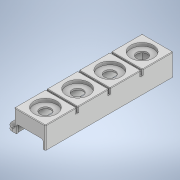
# Autodesk Inventor part: Knob_Base
Saved by Autodesk Inventor 2021 (Build 250183000, 183)
## iProperties
Created: 2020-07-22
Part Number: Knob_Base
Material: Generic
Document SubType Name: Modeling
Designer: ameli
Density: 1 g/cm^3
Appearance: Default
Author: ameli
Autodesk Inventor part; units mm, degrees
ref_plane "YZ Plane" through (0, 0, 0) normal (1, 0, 0) x (0, 1, 0)
ref_plane "XZ Plane" through (0, 0, 0) normal (0, 1, 0) x (-1, 0, 0)
ref_plane "XY Plane" through (0, 0, 0) normal (0, 0, 1) x (1, 0, 0)
sketch "Sketch1" plane through (0, 0, 0) normal (0, 1, 0) x (-1, 0, 0)
  line L0 (14.5, 59.5) -> (-14.5, 59.5)
  line L1 (-14.5, 59.5) -> (-14.5, -59.5)
  line L2 (-14.5, -59.5) -> (14.5, -59.5)
  line L3 (14.5, -59.5) -> (14.5, 59.5)
  point P0 (0, 0)
  dimension "d0" = 119
  dimension "d1" = 29
  dimension "d2" = 14.5
  dimension "d3" = 59.5
  constraints: 8 end point, 2 parallel, 1 horizontal, 1 perpendicular
  measures "d0" distance of L2.end L0.start
  measures "d1" distance of L1.end L2.end
  measures "d2" distance from line of point (0, 0) L3
  measures "d3" distance from line of point (0, 0) L2
extrude "Extrusion1" add sketch "Sketch1" along normal blind 20.3
sketch "Sketch2" plane through (0, 20.3, 0) normal (0, 1, 0) x (1, 0, 0)
  circle A0 centre (0, -45) radius 10.5
  circle A1 centre (0, -15) radius 10.5
  circle A2 centre (0, 15) radius 10.5
  circle A3 centre (0, 45) radius 10.5
  line L0 (-14.5, 59.5) -> (-14.5, -59.5) projected
  line L1 (-14.5, -59.5) -> (14.5, -59.5) projected
  line L2 (14.5, 59.5) -> (-14.5, 59.5) projected
  point P0 (0, 0)
  dimension "d9" = 21
  dimension "d10" = 21
  dimension "d11" = 21
  dimension "d12" = 21
  dimension "d13" = 14.5
  dimension "d14" = 14.5
  dimension "d15" = 14.5
  dimension "d16" = 14.5
  dimension "d17" = 14.5
  dimension "d18" = 14.5
  dimension "d19" = 44.5
  dimension "d20" = 44.5
  constraints: 4 centre point
  measures "d9" diameter of A0
  measures "d10" diameter of A1
  measures "d11" diameter of A2
  measures "d12" diameter of A3
  measures "d13" distance from line of L0 A0.centre
  measures "d14" distance from line of L0 A1.centre
  measures "d15" distance from line of L0 A2.centre
  measures "d16" distance from line of L0 A3.centre
  measures "d17" distance from line of L1 A0.centre
  measures "d18" distance from line of A3.centre L2
  measures "d19" distance from line of L1 A1.centre
  measures "d20" distance from line of L2 A2.centre
extrude "Extrusion2" cut sketch "Sketch2" against normal through all
sketch "Sketch3" plane through (0, 20.3, 0) normal (0, 1, 0) x (1, 0, 0)
  line L0 (-14.5, -30.5) -> (14.5, -30.5)
  line L1 (14.5, -30.5) -> (14.5, -29.5)
  line L2 (14.5, -29.5) -> (-14.5, -29.5)
  line L3 (-14.5, -29.5) -> (-14.5, -30.5)
  line L4 (-14.5, -0.5) -> (14.5, -0.5)
  line L5 (14.5, -0.5) -> (14.5, 0.5)
  line L6 (14.5, 0.5) -> (-14.5, 0.5)
  line L7 (-14.5, 0.5) -> (-14.5, -0.5)
  line L8 (-14.5, 29.5) -> (14.5, 29.5)
  line L9 (14.5, 29.5) -> (14.5, 30.5)
  line L10 (14.5, 30.5) -> (-14.5, 30.5)
  line L11 (-14.5, 30.5) -> (-14.5, 29.5)
  line L12 (-14.5, 59.5) -> (-14.5, -59.5) projected
  line L13 (-14.5, -59.5) -> (14.5, -59.5) projected
  point P0 (0, 0)
  dimension "d23" = 1
  dimension "d24" = 1
  dimension "d25" = 1
  dimension "d26" = 29
  dimension "d27" = 0
  dimension "d28" = 0
  dimension "d29" = 29
  dimension "d30" = 29
  dimension "d31" = 29
  dimension "d32" = 29
  dimension "d33" = 29
  constraints: 24 end point, 6 parallel, 3 horizontal, 3 perpendicular, 1 point on line
  measures "d23" distance of L2.end L0.start
  measures "d24" distance of L6.end L4.start
  measures "d25" distance of L10.end L8.start
  measures "d26" distance of L1.end L2.end
  measures "d27" distance between parallel lines of L12 L3
  measures "d28" distance between parallel lines of L12 L11
  measures "d29" distance of L4.start L4.end
  measures "d30" distance of L8.start L8.end
  measures "d31" distance between parallel lines of L13 L0
  measures "d32" distance between parallel lines of L4 L2
  measures "d33" distance between parallel lines of L8 L6
extrude "Extrusion3" cut sketch "Sketch3" against normal blind 5
shell "Shell2" thickness 1.5 removed faces 5 at (13.1667, 0, -5) at (10.466, 6.7667, 45.8449) at (10.466, 6.7667, 15.8449) at (10.466, 6.7667, -14.1551) at (10.466, 6.7667, -44.1551)
fillet "Fillet3" radius 1 16 edges at (14.5, 10.15, 59.5) (14.5, 10.15, -59.5) (-14.5, 10.15, 59.5) (-14.5, 10.15, -59.5) (14.5, 17.8, -30.5) (14.5, 17.8, -29.5) (14.5, 17.8, 0.5) (14.5, 17.8, -0.5) (14.5, 17.8, 30.5) (14.5, 17.8, 29.5) (-14.5, 17.8, -29.5) (-14.5, 17.8, -30.5) (-14.5, 17.8, 0.5) (-14.5, 17.8, -0.5) (-14.5, 17.8, 30.5) (-14.5, 17.8, 29.5)
fillet "Fillet4" radius 0.5 32 edges at (-14.2071, 20.3, -30.7929) (0, 20.3, -30.5) (14.2071, 20.3, -30.7929) (14.5, 20.3, -45) (14.2071, 20.3, -59.2071) (0, 20.3, -59.5) (-14.2071, 20.3, -59.2071) (-14.5, 20.3, -45) (-14.2071, 20.3, -0.7929) (0, 20.3, -0.5) (14.2071, 20.3, -0.7929) (14.5, 20.3, -15) (14.2071, 20.3, -29.2071) (0, 20.3, -29.5) (-14.2071, 20.3, -29.2071) (-14.5, 20.3, -15) (-14.2071, 20.3, 29.2071) (0, 20.3, 29.5) (14.2071, 20.3, 29.2071) (14.5, 20.3, 15) (14.2071, 20.3, 0.7929) (0, 20.3, 0.5) (-14.2071, 20.3, 0.7929) (-14.5, 20.3, 15) (-14.2071, 20.3, 59.2071) (0, 20.3, 59.5) (14.2071, 20.3, 59.2071) (14.5, 20.3, 45) (14.2071, 20.3, 30.7929) (0, 20.3, 30.5) (-14.2071, 20.3, 30.7929) (-14.5, 20.3, 45)
sketch "Sketch4" plane through (-13.5, 0, 59.5) normal (0, 0, 1) x (1, 0, 0)
  line L0 (1, 8) -> (26, 8)
  line L1 (26, 8) -> (26, 0)
  line L2 (26, 0) -> (1, 0)
  line L3 (1, 0) -> (1, 8)
  line L4 (0, 0) -> (27, 0) projected
  line L5 (-1, 19.8) -> (-1, 0) projected
  line L6 (28, 0) -> (28, 19.8) projected
  point P0 (13.5, 0)
  dimension "d40" = 8
  dimension "d41" = 0
  dimension "d42" = 2
  dimension "d45" = 2
  constraints: 8 end point, 2 parallel, 1 horizontal, 1 perpendicular
  measures "d40" distance of L0.end L1.end
  measures "d41" distance between parallel lines of L4 L2
  measures "d42" distance between parallel lines of L5 L3
  measures "d45" distance between parallel lines of L6 L1
extrude "Extrusion4" cut sketch "Sketch4" against normal blind 2
sketch "Sketch5" plane through (0, 0, 0) normal (0, -1, 0) x (1, 0, 0)
  line L0 (-16.5, -59.5) -> (-13, -59.5)
  line L1 (-13, -59.5) -> (-13, 59.5)
  line L2 (-13, 59.5) -> (-16.5, 59.5)
  line L3 (-21.5, 54.5) -> (-21.5, -54.5)
  line L4 (-13, -58) -> (-13, 58) projected
  line L5 (-12.5, 59.5) -> (12.5, 59.5) projected
  line L6 (13.5, -59.5) -> (-13.5, -59.5) projected
  line L7 (-14.5, 31.5) -> (-14.5, 28.5) projected
  arc A0 (-16.5, 59.5) -> (-21.5, 54.5) centre (-16.5, 54.5) ccw
  arc A1 (-21.5, -54.5) -> (-16.5, -59.5) centre (-16.5, -54.5) ccw
  point P0 (0, 0)
  dimension "d46" = 7
  dimension "d47" = 5
  constraints: 8 end point, 4 point on circle, 4 tangent, 3 collinear, 2 centre point, 2 parallel, 1 equal radius, 1 horizontal, 1 perpendicular
  measures "d46" distance between parallel lines of L7 L3
  measures "d47" radius of A0
extrude "Extrusion5" add sketch "Sketch5" against normal blind 3
sketch "Sketch6" plane through (0, 3, 0) normal (0, 1, 0) x (1, 0, 0)
  line L0 (-21.5, 54.5) -> (-21.5, -54.5) projected
  line L1 (-14.5, 28.5) -> (-14.5, 31.5) projected
  line L2 (-14.5, -31.5) -> (-14.5, -58.5) projected
  line L3 (-14.5, -31.5) -> (-14.5, -28.5) projected
  line L4 (-14.5, -1.5) -> (-14.5, -28.5) projected
  line L5 (-14.5, -1.5) -> (-14.5, 1.5) projected
  line L6 (-14.5, 28.5) -> (-14.5, 1.5) projected
  line L7 (-14.5, 28.5) -> (-14.5, 31.5) projected
  line L8 (-14.5, 58.5) -> (-14.5, 31.5) projected
  line L9 (-16.5, 59.5) -> (13.5, 59.5) projected
  line L10 (-13.5, -59.5) -> (13.5, -59.5) projected
  line L11 (-14.5, 58.5) -> (-14.5, -58.5) projected
  point P0 (0, 0)
  point P1 (-18, -49.5)
  point P2 (-18, 0)
  point P3 (-18, 49.5)
  dimension "d51" = 3.5
  dimension "d52" = 10
  dimension "d53" = 10
  dimension "d54" = 49.5
  constraints: 2 vertical alignment
  measures "d51" distance from line of L0 point (-18, 49.5)
  measures "d52" distance from line of L9 point (-18, 49.5)
  measures "d53" distance from line of point (-18, -49.5) L10
  measures "d54" distance of point (-18, -49.5) point (-18, 0)
hole "Hole1" at (-18, 3, 49.5) at (-18, 3, 0) at (-18, 3, -49.5) direction (0, -1, 0) diameter 3 end through all counterbore diameter 5 counterbore depth 1.5
fillet "Fillet6" radius 2 3 edges at (-14.2071, 3, 59.2071) (-14.2071, 3, -59.2071) (-14.5, 3, 0)
sketch "Sketch7" plane through (-13, 18.8, 32) normal (0, -1, 0) x (1, 0, 0)
  circle A0 centre (13, 13) radius 10.5 projected
  circle A1 centre (13, 13) radius 12.5
  circle A2 centre (13, 13) radius 5
  line L0 (-1, 26.5) -> (-1, -0.5) projected
  circle A3 centre (13, -17) radius 5
  circle A4 centre (13, -17) radius 12.5
  circle A5 centre (13, -47) radius 5
  circle A6 centre (13, -47) radius 12.5
  circle A7 centre (13, -77) radius 5
  circle A8 centre (13, -77) radius 12.5
  circle A9 centre (13, -17) radius 10.5 projected
  point P0 (13, -32)
  dimension "d63" = 2
  dimension "d64" = 10
  dimension "d67" = 30
  constraints: 8 centre point, 4 coincident, 1 vertical, 12 other
  measures "d63" radial gap between concentric circles of A0 A1
  measures "d64" diameter of A2
  measures "d67" distance of A2.centre A3.centre
extrude "Extrusion6" add sketch "Sketch7" along normal blind 3 contours A0 | A1 | A4 | A6 | A8 | A9
sketch "Sketch8" plane through (0, 18.8, -45) normal (0, 1, 0) x (1, 0, 0)
  circle A0 centre (0, 0) radius 10.5 projected
  circle A1 centre (0, -30) radius 10.5 projected
  circle A2 centre (0, -60) radius 10.5 projected
  circle A3 centre (0, -90) radius 10.5 projected
  point P0 (0, -45)
extrude "Extrusion7" cut sketch "Sketch8" against normal blind 1.5
fillet "Fillet7" radius 2 2 edges at (12.5, 8, 58.75) (-12.5, 8, 58.75)
body "Solid1"
